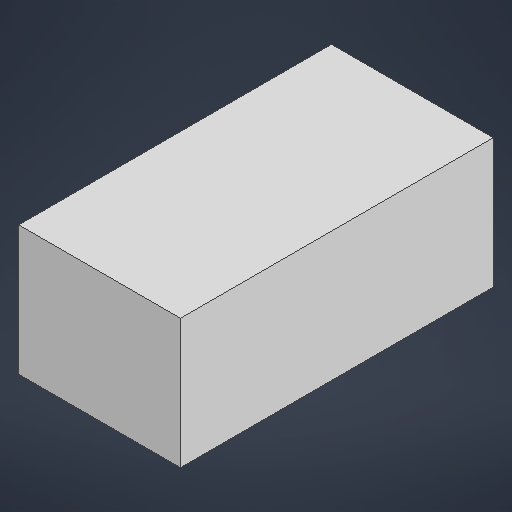
# Autodesk Inventor part: NRF24L01+
Saved by Autodesk Inventor 2026.1 (Build 301233000, 233)
## iProperties
Created: 2026-07-05
Part Number: NRF24L01+
Material: Generic
Document SubType Name: Modeling
Designer: Kasi Pusuluri
Density: 1 g/cm^3
Appearance: Default
Author: Kasi Pusuluri
Autodesk Inventor part; units mm, degrees
ref_plane "YZ Plane" through (0, 0, 0) normal (1, 0, 0) x (0, 1, 0)
ref_plane "XZ Plane" through (0, 0, 0) normal (0, 1, 0) x (-1, 0, 0)
ref_plane "XY Plane" through (0, 0, 0) normal (0, 0, 1) x (1, 0, 0)
sketch "Sketch1" plane through (0, 0, 0) normal (0, 1, 0) x (-1, 0, 0)
  line L0 (0, 0) -> (15, 0)
  line L1 (15, 0) -> (15, -29)
  line L2 (15, -29) -> (0, -29)
  line L3 (0, -29) -> (0, 0)
  dimension "d0" = 15
  dimension "d1" = 29
  constraints: 8 end point, 2 parallel, 1 horizontal, 1 perpendicular
  measures "d0" distance of L1.end L2.end
  measures "d1" distance of L0.end L1.end
extrude "Extrusion1" add sketch "Sketch1" along normal blind 12
body "Solid1"
